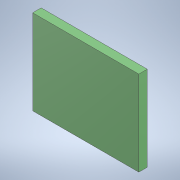
# Autodesk Inventor part: placa-circuito
Saved by Autodesk Inventor 2021 (Build 250183000, 183)
## iProperties
Created: 2023-11-09
Part Number: placa-circuito
Material: Genérico
Document SubType Name: Modeling
Designer: Vinicius
Density: 1 g/cm^3
Appearance: Padrão
Author: Vinicius
Autodesk Inventor part; units mm, degrees
ref_plane "YZ Plane" through (0, 0, 0) normal (1, 0, 0) x (0, 1, 0)
ref_plane "XZ Plane" through (0, 0, 0) normal (0, 1, 0) x (-1, 0, 0)
ref_plane "XY Plane" through (0, 0, 0) normal (0, 0, 1) x (1, 0, 0)
sketch "Esboço1" plane through (0, 0, 0) normal (0, 0, 1) x (1, 0, 0)
  line L0 (-125, -100) -> (125, -100)
  line L1 (125, -100) -> (125, 100)
  line L2 (125, 100) -> (-125, 100)
  line L3 (-125, 100) -> (-125, -100)
  line L4 (-125, -100) -> (125, 100) construction
  line L5 (125, -100) -> (-125, 100) construction
  point P0 (0, 0)
  dimension "d0" = 200
  dimension "d1" = 250
  constraints: 12 end point, 2 midpoint, 2 parallel, 1 horizontal, 1 perpendicular
  measures "d0" distance of L2.end L0.start
  measures "d1" distance of L0.start L0.end
extrude "Extrusão1" add sketch "Esboço1" along normal blind 20
